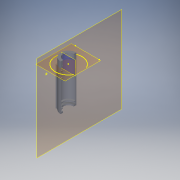
# Autodesk Inventor part: 12_Lenstube
Saved by Autodesk Inventor 2016 (Build 200138000, 138)
## iProperties
Created: 2016-11-01
Part Number: 12_Lenstube
Material: Generisch
Document SubType Name: Modeling
Designer: Bene
Density: 1 g/cm^3
Appearance: Vorgabe
Author: Bene
Autodesk Inventor part; units mm, degrees
ref_plane "YZ Plane" through (0, 0, 0) normal (1, 0, 0) x (0, 1, 0)
ref_plane "XZ Plane" through (0, 0, 0) normal (0, 1, 0) x (-1, 0, 0)
ref_plane "XY Plane" through (0, 0, 0) normal (0, 0, 1) x (1, 0, 0)
ref_plane "Arbeitsebene1" through (0, 0, 0) normal (0, 0, 1) x (1, 0, 0)
sketch "Skizze1" plane through (0, 0, 0) normal (0, 0, 1) x (1, 0, 0)
  arc A0 (0, -20.5627) -> (0, -40.4373) centre (-18.5, -30.5) ccw projected
  point P0 (0, 0)
ref_plane "Arbeitsebene2" through (-18.5, -30.5, 0) normal (0, 1, 0) x (-1, 0, 0)
sketch "Skizze2" plane through (-18.5, -30.5, 0) normal (0, 1, 0) x (-1, 0, 0)
  line L0 (-0.0002, 0) -> (-0.0002, -109.9299) construction
  line L1 (-18.5, 4.7902) -> (0.0006, 4.7902) construction
  line L2 (-18.5, -58.2098) -> (-0.0002, -58.2098) construction
  line L3 (-11.0002, -59.4598) -> (10.9998, -59.4598) construction
  line L4 (10.9998, -59.4598) -> (10.9998, -56.9598)
  line L5 (10.9998, -56.9598) -> (-11.0002, -56.9598) construction
  line L6 (-11.0002, -56.9598) -> (-11.0002, -59.4598)
  line L7 (-11.0002, -59.4598) -> (10.9998, -56.9598) construction
  line L8 (10.9998, -59.4598) -> (-11.0002, -56.9598) construction
  arc A0 (10.9998, -56.9598) -> (-11.0002, -56.9598) centre (-0.0002, -105.7348) ccw
  arc A1 (-11.0002, -59.4598) -> (10.9998, -59.4598) centre (-0.0002, -10.6848) ccw
  line L9 (-9.1994, 7.5402) -> (9.2006, 7.5402) construction
  line L10 (9.2006, 7.5402) -> (9.2006, 2.0402)
  line L11 (9.2006, 2.0402) -> (-9.1994, 2.0402) construction
  line L12 (-9.1994, 2.0402) -> (-9.1994, 7.5402)
  line L13 (-9.1994, 7.5402) -> (9.2006, 2.0402) construction
  line L14 (9.2006, 7.5402) -> (-9.1994, 2.0402) construction
  arc A2 (-9.1994, 2.0402) -> (9.2006, 2.0402) centre (0.0006, 40.9678) ccw
  arc A3 (9.2006, 7.5402) -> (-9.1994, 7.5402) centre (0.0006, -31.3875) ccw
  line L15 (11.1987, -59.5944) -> (11.1988, -56.7897)
  line L16 (-11.2001, -56.8002) -> (-11.2001, -59.6195)
  line L17 (9.4006, 1.8822) -> (9.3977, 7.6862)
  arc A4 (9.3977, 7.6862) -> (8.4813, 7.8953) centre (0.0006, -31.3875) ccw
  line L18 (-9.4014, 7.6981) -> (-9.3986, 1.8822)
  arc A5 (8.4813, 1.6725) -> (9.4006, 1.8822) centre (0.0006, 40.9678) ccw
  line L19 (8.4813, 1.6725) -> (65.1172, 1.6725) construction
  arc A6 (11.1988, -56.7897) -> (8.4813, -56.2464) centre (-0.0002, -105.7348) ccw
  arc A7 (-0.0002, -55.5348) -> (-11.2001, -56.8002) centre (-0.0002, -105.7348) ccw
  line L20 (8.4813, -60.1381) -> (8.4813, -62.3532)
  line L21 (8.4813, -60.1381) -> (10.6964, -60.1381) construction
  line L22 (8.4813, -62.3532) -> (12.4, -62.3532)
  line L23 (12.4, -62.3532) -> (12.4, 9.6468)
  line L24 (12.4, 9.6468) -> (8.4813, 9.6468)
  line L25 (8.4813, 9.6468) -> (8.4813, 7.8953)
  line L26 (8.4813, 1.6725) -> (8.4813, 0.6725)
  line L27 (8.4813, 0.6725) -> (11.3792, 0.6725)
  line L28 (11.3792, 0.6725) -> (11.3792, -55.3275)
  line L29 (11.3792, -55.3275) -> (8.4813, -55.3275)
  line L30 (8.4813, -55.3275) -> (8.4813, -56.2464)
  arc A8 (-11.2001, -59.6195) -> (-0.0002, -60.8848) centre (-0.0002, -10.6848) ccw
  arc A9 (8.4813, -60.1381) -> (11.1987, -59.5944) centre (-0.0002, -10.6848) ccw
  point P0 (-18.5, 0)
  dimension "d0" = 22
  dimension "d1" = 2.5
  dimension "d2" = 50
  dimension "d3" = 50
  dimension "d4" = 18.4
  dimension "d5" = 5.5
  dimension "d6" = 40
  dimension "d7" = 40
  dimension "d9" = 0.2
  dimension "d12" = 90
  dimension "d14" = 72
  dimension "d15" = 90
  dimension "d17" = 56
  dimension "d18" = 0
  constraints: 62 end point, 20 point on circle, 11 perpendicular, 10 centre point, 6 parallel, 6 point on line, 5 horizontal, 4 midpoint, 2 vertical
  measures "d0" distance of L5.end L4.end
  measures "d1" distance of L4.end L3.end
  measures "d2" radius of A0
  measures "d3" radius of A1
  measures "d4" distance of L10.end L11.end
  measures "d5" distance of L9.end L10.end
  measures "d6" radius of A2
  measures "d7" radius of A3
  measures "d9" radial gap between concentric circles of A2 A5
  measures "d12" angle of L20 L21
  measures "d14" distance of L22.end L23.end
  measures "d15" angle of L23 L22
  measures "d17" distance of L27.end L28.end
  measures "d18" distance between parallel lines of L20 L30
revolve "Umdrehung1" add sketch "Skizze2" angle 180 mid plane about axis through (-18.4998, -30.5, 0) along (0, 0, -1) contours L15 A6 L30 L29 L28 L27 L26 A5 L17 A4 L25 L24 L23 L22 L20 A9
ref_plane "Arbeitsebene3" through (-38, 7.1361, -57.0623) normal (1, 0, 0) x (0, 0, -1)
sketch "Skizze3" plane through (-38, 7.1361, -57.0623) normal (1, 0, 0) x (0, 0, -1)
  circle A0 centre (-41.5623, -19.6361) radius 1.5 construction
  circle A1 centre (-41.5623, -53.1361) radius 1.5 construction
  point P0 (-57.0623, -7.1361)
sketch "Skizze5" plane through (-18.4998, -42.9002, -62.3532) normal (0, 0, -1) x (-1, 0, 0)
  arc A0 (0, 0) -> (0, 24.8003) centre (0, 12.4002) ccw projected
  arc A1 (0, 0) -> (0, 24.8003) centre (0, 12.4002) ccw projected
  line L0 (12.4002, 12.4002) -> (9.4744, 12.4002)
  line L1 (9.4744, 12.4002) -> (9.4744, 20.4002)
  line L2 (9.4744, 20.4002) -> (12.4002, 20.4002)
  line L3 (12.4002, 20.4002) -> (12.4002, 12.4002)
  line L4 (12.4002, 12.4002) -> (9.4744, 12.4002)
  line L5 (9.4744, 12.4002) -> (9.4744, 4.4002)
  line L6 (9.4744, 4.4002) -> (12.4002, 4.4002)
  line L7 (12.4002, 4.4002) -> (12.4002, 12.4002)
  point P0 (-18.4998, 42.9002)
  dimension "d27" = 8
  dimension "d28" = 8
  constraints: 16 end point, 4 parallel, 4 point on circle, 2 horizontal, 2 perpendicular
  measures "d27" distance of L0.end L1.end
  measures "d28" distance of L5.end L4.end
extrude "Extrusion2" add sketch "Skizze5" against normal blind 60 contours A0 L7 L6 | A0 L2 L3
fillet "Rundung1" radius 4 2 edges at (-27.9742, -38.5, -32.3532) (-27.9742, -22.5, -32.3532)
sketch "Skizze4" plane through (-18.4998, -22.0185, -62.3532) normal (1, 0, 0) x (0, 0, -1)
  line L0 (-5.5634, 2.7174) -> (-2.7588, 2.7174) projected
  arc A0 (-2.2151, 0) -> (-2.7588, 2.7174) centre (-51.6683, -8.4815) ccw projected
  line L1 (-2.2151, 0) -> (0, 0) projected
  line L2 (0, 0) -> (0, 3.9187) projected
  line L3 (0, 3.9187) -> (-72, 3.9187) projected
  line L4 (-72, 3.9187) -> (-72, 0) projected
  line L5 (-72, 0) -> (-70.2485, 0) projected
  arc A1 (-70.0394, 0.9164) -> (-70.2485, 0) centre (-30.9657, -8.4807) ccw projected
  line L6 (-70.0394, 0.9164) -> (-64.2354, 0.9193) projected
  arc A2 (-64.0257, 0) -> (-64.2354, 0.9193) centre (-103.321, -8.4807) ccw projected
  line L7 (-64.0257, 0) -> (-63.0257, 0) projected
  line L8 (-63.0257, 0) -> (-63.0257, 2.8979) projected
  line L9 (-63.0257, 2.8979) -> (-7.0257, 2.8979) projected
  line L10 (-7.0257, 2.8979) -> (-7.0257, 0) projected
  line L11 (-7.0257, 0) -> (-6.1068, 0) projected
  arc A3 (-5.5634, 2.7174) -> (-6.1068, 0) centre (43.3816, -8.4815) ccw projected
  line L12 (-2.7588, -19.6804) -> (-5.5634, -19.6804) projected
  arc A4 (-6.1068, -16.963) -> (-5.5634, -19.6804) centre (43.3816, -8.4815) ccw projected
  line L13 (-6.1068, -16.963) -> (-7.0257, -16.963) projected
  line L14 (-7.0257, -16.963) -> (-7.0257, -19.8609) projected
  line L15 (-7.0257, -19.8609) -> (-63.0257, -19.8609) projected
  line L16 (-63.0257, -19.8609) -> (-63.0257, -16.963) projected
  line L17 (-63.0257, -16.963) -> (-64.0257, -16.963) projected
  arc A5 (-64.2354, -17.8822) -> (-64.0257, -16.963) centre (-103.321, -8.4822) ccw projected
  line L18 (-64.2354, -17.8822) -> (-70.0394, -17.8794) projected
  arc A6 (-70.2485, -16.963) -> (-70.0394, -17.8794) centre (-30.9657, -8.4822) ccw projected
  line L19 (-70.2485, -16.963) -> (-72, -16.963) projected
  line L20 (-72, -16.963) -> (-72, -20.8816) projected
  line L21 (-72, -20.8816) -> (0, -20.8816) projected
  line L22 (0, -20.8816) -> (0, -16.963) projected
  line L23 (0, -16.963) -> (-2.2151, -16.963) projected
  arc A7 (-2.7588, -19.6804) -> (-2.2151, -16.963) centre (-51.6683, -8.4815) ccw projected
  line L24 (-46.7833, 9.535) -> (-46.7833, -24.0923) construction
  circle A8 centre (-46.7833, -8.4815) radius 2
  circle A9 centre (-56.7833, -8.4815) radius 2
  circle A10 centre (-36.7833, -8.4815) radius 2
  point P0 (-62.3532, 22.0185)
  dimension "d20" = 4
  dimension "d21" = 4
  dimension "d22" = 4
  dimension "d23" = 10
  dimension "d24" = 10
  constraints: 3 centre point, 2 end point, 1 perpendicular, 1 point on line
  measures "d20" diameter of A8
  measures "d21" diameter of A9
  measures "d22" diameter of A10
  measures "d23" distance of A10.centre A8.centre
  measures "d24" distance of A9.centre A8.centre
extrude "Extrusion1" cut sketch "Skizze4" against normal through all contours A8 | A9 | A10
